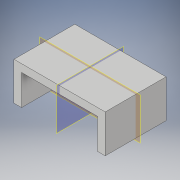
# Autodesk Inventor part: wirebridge2
Saved by Autodesk Inventor 2017 (Build 210142000, 142)
## iProperties
Created: 2018-01-06
Part Number: wirebridge2
Material: Generic
Document SubType Name: Modeling
Designer: Delta
Density: 1 g/cm^3
Appearance: Default
Author: Delta
Autodesk Inventor part; units mm, degrees
ref_plane "YZ Plane" through (0, 0, 0) normal (1, 0, 0) x (0, 1, 0)
ref_plane "XZ Plane" through (0, 0, 0) normal (0, 1, 0) x (-1, 0, 0)
ref_plane "XY Plane" through (0, 0, 0) normal (0, 0, 1) x (1, 0, 0)
sketch "Sketch1" plane through (0, 0, 0) normal (0, 0, 1) x (1, 0, 0)
  line L0 (0, 0) -> (76.2, 0)
  line L1 (76.2, 0) -> (76.2, 31.75)
  line L2 (76.2, 31.75) -> (0, 31.75)
  line L3 (0, 31.75) -> (0, 0)
  line L4 (6.35, 0) -> (69.85, 0)
  line L5 (69.85, 0) -> (69.85, 25.4)
  line L6 (69.85, 25.4) -> (6.35, 25.4)
  line L7 (6.35, 25.4) -> (6.35, 0)
  dimension "d0" = 6.35
  dimension "d1" = 6.35
  dimension "d2" = 6.35
  dimension "d3" = 63.5
  dimension "d4" = 31.75
  constraints: 16 end point, 4 parallel, 2 horizontal, 2 perpendicular, 1 point on line
  measures "d0" distance between parallel lines of L1 L5
  measures "d1" distance between parallel lines of L3 L7
  measures "d2" distance between parallel lines of L2 L6
  measures "d3" distance of L5.end L6.end
  measures "d4" distance between parallel lines of L0 L2
extrude "Extrusion1" add sketch "Sketch1" along normal blind 50.8 contours L3 L2 L1 L0 L5 L6 L7
sketch "Sketch2" plane through (0, 0, 0) normal (0, -1, 0) x (1, 0, 0)
  point P0 (0, 0)
ref_plane "Work Plane1" through (0, 0, 25.4) normal (0, 0, 1) x (1, 0, 0)
ref_plane "Work Plane2" through (38.1, 0, 0) normal (-1, 0, 0) x (0, 0, 1)
sketch "Sketch3" plane through (0, 0, 0) normal (0, -1, 0) x (1, 0, 0)
  circle A0 centre (3.175, 44.45) radius 1.651
  line L0 (0, 50.8) -> (6.35, 50.8) projected
  line L1 (6.35, 0) -> (6.35, 50.8) projected
  line L2 (0, 25.4) -> (76.2, 25.4)
  line L3 (76.2, 0) -> (76.2, 50.8) projected
  circle A1 centre (3.175, 6.35) radius 1.651
  line L4 (38.1, 50.8) -> (38.1, 0)
  circle A2 centre (73.025, 6.35) radius 1.651
  circle A3 centre (73.025, 44.45) radius 1.651
  point P0 (0, 0)
  dimension "d7" = 3.302
  dimension "d8" = 6.35
  dimension "d9" = 3.175
  constraints: 4 centre point, 4 end point, 3 symmetric about line, 1 midpoint, 1 vertical, 3 other
  measures "d7" diameter of A0
  measures "d8" distance from line of L0 A0.centre
  measures "d9" distance from line of L1 A0.centre
extrude "Extrusion2" cut sketch "Sketch3" against normal blind 12.7
body "Solid1"
